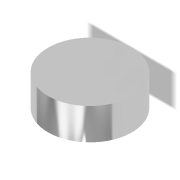
# Autodesk Inventor part: 00_NeoDymMagnet_8x3mm
Saved by Autodesk Inventor 2022 (Build 260153000, 153)
## iProperties
Created: 2022-09-19
Part Number: 00_NeoDymMagnet_8x3mm
Material: Generisch
Document SubType Name: Modeling
Designer: UC2
Density: 1 g/cm^3
Appearance: Chrom - poliert
Author: UC2
Autodesk Inventor part; units mm, degrees
ref_plane "YZ Plane" through (0, 0, 0) normal (1, 0, 0) x (0, 1, 0)
ref_plane "XZ Plane" through (0, 0, 0) normal (0, 1, 0) x (-1, 0, 0)
ref_plane "XY Plane" through (0, 0, 0) normal (0, 0, 1) x (1, 0, 0)
sketch "Skizze1" plane through (0, 0, 0) normal (0, 1, 0) x (-1, 0, 0)
  circle A0 centre (-56.5072, 0) radius 4
  point P0 (0, 0)
  dimension "d0" = 8
  dimension "d0" = 8
  constraints: 1 centre point
  measures "d0" diameter of A0
extrude "Extrusion1" add sketch "Skizze1" along normal blind 3
